Autodesk Inventor part; units mm, degrees
(part 2 of 2)
  spline S121 degree 2 poles (15.6602, 13.1424) (15.6885, 13.0846) (15.7439, 12.8774) (15.7439, 12.7846) knots 0 0 0 1 2 2 2
  spline S122 degree 2 poles (15.7439, 12.7846) (15.7439, 12.5888) (15.5368, 12.368) (15.3602, 12.368) knots 0 0 0 1 2 2 2
  spline S123 degree 2 poles (15.3602, 12.368) (15.2775, 12.368) (15.1394, 12.4065) (15.0805, 12.4405) knots 0 0 0 1 2 2 2
  spline S124 degree 2 poles (15.0805, 12.4405) (15.0194, 12.4744) (14.8994, 12.5729) (14.8417, 12.6273) knots 0 0 0 1 2 2 2
  spline S125 degree 2 poles (14.8417, 12.6273) (14.7454, 12.7156) (14.5394, 12.9318) (14.4794, 12.9963) knots 0 0 0 1 2 2 2
  line L109 (14.4794, 12.9963) -> (14.4794, 12.3103)
  line L110 (14.4794, 12.3103) -> (14.3175, 12.3103)
  line L111 (14.7975, 11.2246) -> (14.7975, 11.391)
  line L112 (14.7975, 11.391) -> (14.3175, 11.391)
  line L113 (14.3175, 11.391) -> (14.3175, 11.571)
  line L114 (14.3175, 11.571) -> (14.7975, 11.571)
  line L115 (14.7975, 11.571) -> (14.7975, 12.188)
  line L116 (14.7975, 12.188) -> (14.9945, 12.188)
  line L117 (14.9945, 12.188) -> (15.7145, 11.5631)
  line L118 (15.7145, 11.5631) -> (15.7145, 11.391)
  line L119 (15.7145, 11.391) -> (14.9481, 11.391)
  line L120 (14.9481, 11.391) -> (14.9481, 11.2246)
  line L121 (14.9481, 11.2246) -> (14.7975, 11.2246)
  line L122 (14.9481, 11.571) -> (15.4937, 11.571)
  line L123 (15.4937, 11.571) -> (14.9481, 12.0408)
  line L124 (14.9481, 12.0408) -> (14.9481, 11.571)
  spline S126 degree 2 poles (14.7613, 10.2284) (14.6605, 10.2284) (14.4884, 10.2929) (14.425, 10.3518) knots 0 0 0 1 2 2 2
  spline S127 degree 2 poles (14.425, 10.3518) (14.3616, 10.4106) (14.2881, 10.5861) (14.2881, 10.6948) knots 0 0 0 1 2 2 2
  spline S128 degree 2 poles (14.2881, 10.6948) (14.2881, 10.7944) (14.3322, 10.9891) (14.3673, 11.0604) knots 0 0 0 1 2 2 2
  line L125 (14.3673, 11.0604) -> (14.5654, 11.0604)
  line L126 (14.5654, 11.0604) -> (14.5654, 11.0469)
  spline S129 degree 2 poles (14.5654, 11.0469) (14.5496, 11.0253) (14.5088, 10.945) (14.4907, 10.8963) knots 0 0 0 1 2 2 2
  spline S130 degree 2 poles (14.4907, 10.8963) (14.4715, 10.8408) (14.4499, 10.7491) (14.4499, 10.6914) knots 0 0 0 1 2 2 2
  spline S131 degree 2 poles (14.4499, 10.6914) (14.4499, 10.6348) (14.4907, 10.5284) (14.5349, 10.4899) knots 0 0 0 1 2 2 2
  spline S132 degree 2 poles (14.5349, 10.4899) (14.5767, 10.4548) (14.6877, 10.4185) (14.7624, 10.4185) knots 0 0 0 1 2 2 2
  spline S133 degree 2 poles (14.7624, 10.4185) (14.8371, 10.4185) (14.9322, 10.4593) (14.9639, 10.4978) knots 0 0 0 1 2 2 2
  spline S134 degree 2 poles (14.9639, 10.4978) (14.999, 10.5374) (15.0284, 10.6552) (15.0284, 10.7265) knots 0 0 0 1 2 2 2
  spline S135 degree 2 poles (15.0284, 10.7265) (15.0284, 10.8035) (15.0047, 10.9563) (14.9945, 11.0027) knots 0 0 0 1 2 2 2
  line L127 (14.9945, 11.0027) -> (15.7145, 11.0027)
  line L128 (15.7145, 11.0027) -> (15.7145, 10.2363)
  line L129 (15.7145, 10.2363) -> (15.5503, 10.2363)
  line L130 (15.5503, 10.2363) -> (15.5503, 10.8227)
  line L131 (15.5503, 10.8227) -> (15.1779, 10.8227)
  spline S136 degree 2 poles (15.1779, 10.8227) (15.1824, 10.7887) (15.1858, 10.7231) (15.1858, 10.6959) knots 0 0 0 1 2 2 2
  spline S137 degree 2 poles (15.1858, 10.6959) (15.1858, 10.5884) (15.1507, 10.4401) (15.0986, 10.3721) knots 0 0 0 1 2 2 2
  spline S138 degree 2 poles (15.0986, 10.3721) (15.0466, 10.3031) (14.8881, 10.2284) (14.7613, 10.2284) knots 0 0 0 1 2 2 2
  spline S139 degree 2 poles (14.7703, 9.1438) (14.6628, 9.1438) (14.4805, 9.2151) (14.4194, 9.2751) knots 0 0 0 1 2 2 2
  spline S140 degree 2 poles (14.4194, 9.2751) (14.3549, 9.3374) (14.2881, 9.4936) (14.2881, 9.5876) knots 0 0 0 1 2 2 2
  spline S141 degree 2 poles (14.2881, 9.5876) (14.2881, 9.6816) (14.3515, 9.8367) (14.4149, 9.8955) knots 0 0 0 1 2 2 2
  spline S142 degree 2 poles (14.4149, 9.8955) (14.4907, 9.968) (14.7454, 10.0495) (14.9311, 10.0495) knots 0 0 0 1 2 2 2
  spline S143 degree 2 poles (14.9311, 10.0495) (15.1134, 10.0495) (15.4066, 9.9748) (15.5152, 9.8967) knots 0 0 0 1 2 2 2
  spline S144 degree 2 poles (15.5152, 9.8967) (15.6217, 9.8208) (15.7405, 9.5808) (15.7405, 9.4234) knots 0 0 0 1 2 2 2
  spline S145 degree 2 poles (15.7405, 9.4234) (15.7405, 9.377) (15.7315, 9.2955) (15.7213, 9.2649) knots 0 0 0 1 2 2 2
  line L132 (15.7213, 9.2649) -> (15.5413, 9.2649)
  line L133 (15.5413, 9.2649) -> (15.5413, 9.2729)
  spline S146 degree 2 poles (15.5413, 9.2729) (15.5549, 9.2989) (15.5786, 9.394) (15.5786, 9.4483) knots 0 0 0 1 2 2 2
  spline S147 degree 2 poles (15.5786, 9.4483) (15.5786, 9.6227) (15.3432, 9.8367) (15.1122, 9.857) knots 0 0 0 1 2 2 2
  spline S148 degree 2 poles (15.1122, 9.857) (15.1586, 9.7902) (15.2096, 9.6499) (15.2096, 9.5661) knots 0 0 0 1 2 2 2
  spline S149 degree 2 poles (15.2096, 9.5661) (15.2096, 9.4846) (15.1768, 9.3623) (15.1269, 9.2955) knots 0 0 0 1 2 2 2
  spline S150 degree 2 poles (15.1269, 9.2955) (15.0692, 9.2185) (14.8903, 9.1438) (14.7703, 9.1438) knots 0 0 0 1 2 2 2
  spline S151 degree 2 poles (14.7624, 9.334) (14.8484, 9.334) (14.9651, 9.3793) (15.0058, 9.4291) knots 0 0 0 1 2 2 2
  spline S152 degree 2 poles (15.0058, 9.4291) (15.0352, 9.4665) (15.0545, 9.5593) (15.0545, 9.608) knots 0 0 0 1 2 2 2
  spline S153 degree 2 poles (15.0545, 9.608) (15.0545, 9.6736) (15.0149, 9.797) (14.9775, 9.857) knots 0 0 0 1 2 2 2
  spline S154 degree 2 poles (14.9775, 9.857) (14.9571, 9.8582) (14.9186, 9.8604) (14.8892, 9.8604) knots 0 0 0 1 2 2 2
  spline S155 degree 2 poles (14.8892, 9.8604) (14.7443, 9.8604) (14.5666, 9.8038) (14.5201, 9.7608) knots 0 0 0 1 2 2 2
  spline S156 degree 2 poles (14.5201, 9.7608) (14.476, 9.7212) (14.4409, 9.6351) (14.4409, 9.5865) knots 0 0 0 1 2 2 2
  spline S157 degree 2 poles (14.4409, 9.5865) (14.4409, 9.4733) (14.6016, 9.334) (14.7624, 9.334) knots 0 0 0 1 2 2 2
  line L134 (15.5051, 8.1012) -> (14.3175, 8.7057)
  line L135 (14.3175, 8.7057) -> (14.3175, 8.9049)
  line L136 (14.3175, 8.9049) -> (15.5503, 8.2664)
  line L137 (15.5503, 8.2664) -> (15.5503, 8.9876)
  line L138 (15.5503, 8.9876) -> (15.7145, 8.9876)
  line L139 (15.7145, 8.9876) -> (15.7145, 8.1012)
  line L140 (15.7145, 8.1012) -> (15.5051, 8.1012)
  spline S158 degree 2 poles (15.016, 7.0608) (14.6401, 7.0608) (14.2881, 7.2793) (14.2881, 7.5068) knots 0 0 0 1 2 2 2
  spline S159 degree 2 poles (14.2881, 7.5068) (14.2881, 7.7378) (14.6469, 7.954) (15.0149, 7.954) knots 0 0 0 1 2 2 2
  spline S160 degree 2 poles (15.0149, 7.954) (15.393, 7.954) (15.7428, 7.7355) (15.7428, 7.5068) knots 0 0 0 1 2 2 2
  spline S161 degree 2 poles (15.7428, 7.5068) (15.7428, 7.277) (15.3805, 7.0608) (15.016, 7.0608) knots 0 0 0 1 2 2 2
  spline S162 degree 2 poles (14.5903, 7.3008) (14.6594, 7.2736) (14.8722, 7.251) (15.016, 7.251) knots 0 0 0 1 2 2 2
  spline S163 degree 2 poles (15.016, 7.251) (15.1598, 7.251) (15.3715, 7.2736) (15.4428, 7.3019) knots 0 0 0 1 2 2 2
  spline S164 degree 2 poles (15.4428, 7.3019) (15.5141, 7.3302) (15.5877, 7.4287) (15.5877, 7.5068) knots 0 0 0 1 2 2 2
  spline S165 degree 2 poles (15.5877, 7.5068) (15.5877, 7.5849) (15.5141, 7.6857) (15.4405, 7.7151) knots 0 0 0 1 2 2 2
  spline S166 degree 2 poles (15.4405, 7.7151) (15.3692, 7.7434) (15.1518, 7.7638) (15.0149, 7.7638) knots 0 0 0 1 2 2 2
  spline S167 degree 2 poles (15.0149, 7.7638) (14.8677, 7.7638) (14.6707, 7.7457) (14.5937, 7.7162) knots 0 0 0 1 2 2 2
  spline S168 degree 2 poles (14.5937, 7.7162) (14.5213, 7.6891) (14.4432, 7.5883) (14.4432, 7.5068) knots 0 0 0 1 2 2 2
  spline S169 degree 2 poles (14.4432, 7.5068) (14.4432, 7.4298) (14.5167, 7.3291) (14.5903, 7.3008) knots 0 0 0 1 2 2 2
  spline S170 degree 2 poles (15.582, 6.5049) (15.582, 6.5559) (15.5571, 6.6566) (15.5379, 6.7053) knots 0 0 0 1 2 2 2
  spline S171 degree 2 poles (15.5379, 6.7053) (15.5186, 6.7506) (15.4779, 6.8174) (15.4598, 6.8434) knots 0 0 0 1 2 2 2
  line L141 (15.4598, 6.8434) -> (15.4598, 6.8547)
  line L142 (15.4598, 6.8547) -> (15.6579, 6.8547)
  spline S172 degree 2 poles (15.6579, 6.8547) (15.6907, 6.7936) (15.7439, 6.5842) (15.7439, 6.4902) knots 0 0 0 1 2 2 2
  spline S173 degree 2 poles (15.7439, 6.4902) (15.7439, 6.3951) (15.7054, 6.2536) (15.6647, 6.1958) knots 0 0 0 1 2 2 2
  spline S174 degree 2 poles (15.6647, 6.1958) (15.6205, 6.1347) (15.4926, 6.0713) (15.4066, 6.0713) knots 0 0 0 1 2 2 2
  spline S175 degree 2 poles (15.4066, 6.0713) (15.2911, 6.0713) (15.1168, 6.223) (15.0941, 6.3294) knots 0 0 0 1 2 2 2
  line L143 (15.0941, 6.3294) -> (15.0805, 6.3294)
  spline S176 degree 2 poles (15.0805, 6.3294) (15.0715, 6.2853) (15.0307, 6.1845) (14.99, 6.1415) knots 0 0 0 1 2 2 2
  spline S177 degree 2 poles (14.99, 6.1415) (14.9503, 6.0985) (14.8235, 6.0441) (14.7318, 6.0441) knots 0 0 0 1 2 2 2
  spline S178 degree 2 poles (14.7318, 6.0441) (14.6379, 6.0441) (14.4783, 6.1087) (14.4171, 6.1675) knots 0 0 0 1 2 2 2
  spline S179 degree 2 poles (14.4171, 6.1675) (14.3537, 6.2287) (14.2881, 6.4019) (14.2881, 6.5117) knots 0 0 0 1 2 2 2
  spline S180 degree 2 poles (14.2881, 6.5117) (14.2881, 6.617) (14.339, 6.823) (14.3741, 6.8932) knots 0 0 0 1 2 2 2
  line L144 (14.3741, 6.8932) -> (14.5722, 6.8932)
  line L145 (14.5722, 6.8932) -> (14.5722, 6.8796)
  spline S181 degree 2 poles (14.5722, 6.8796) (14.5292, 6.8208) (14.4499, 6.6215) (14.4499, 6.523) knots 0 0 0 1 2 2 2
  spline S182 degree 2 poles (14.4499, 6.523) (14.4499, 6.4653) (14.4862, 6.3498) (14.5281, 6.3113) knots 0 0 0 1 2 2 2
  spline S183 degree 2 poles (14.5281, 6.3113) (14.57, 6.274) (14.6696, 6.2343) (14.7454, 6.2343) knots 0 0 0 1 2 2 2
  spline S184 degree 2 poles (14.7454, 6.2343) (14.8213, 6.2343) (14.9198, 6.2785) (14.9481, 6.3181) knots 0 0 0 1 2 2 2
  spline S185 degree 2 poles (14.9481, 6.3181) (14.9764, 6.3577) (14.9979, 6.4653) (14.9979, 6.5287) knots 0 0 0 1 2 2 2
  line L146 (14.9979, 6.5287) -> (14.9979, 6.6079)
  line L147 (14.9979, 6.6079) -> (15.153, 6.6079)
  line L148 (15.153, 6.6079) -> (15.153, 6.5457)
  spline S186 degree 2 poles (15.153, 6.5457) (15.153, 6.42) (15.273, 6.2615) (15.3873, 6.2615) knots 0 0 0 1 2 2 2
  spline S187 degree 2 poles (15.3873, 6.2615) (15.4405, 6.2615) (15.5164, 6.3023) (15.539, 6.3351) knots 0 0 0 1 2 2 2
  spline S188 degree 2 poles (15.539, 6.3351) (15.5628, 6.3702) (15.582, 6.4562) (15.582, 6.5049) knots 0 0 0 1 2 2 2
  line L149 (12.0174, 19.3553) -> (12.0174, 19.5319)
  line L150 (12.0174, 19.5319) -> (12.1238, 19.5319)
  spline S189 degree 2 poles (12.1238, 19.5319) (12.0898, 19.5726) (12.0445, 19.6326) (12.0253, 19.6734) knots 0 0 0 1 2 2 2
  spline S190 degree 2 poles (12.0253, 19.6734) (12.0072, 19.7107) (11.9879, 19.7911) (11.9879, 19.8443) knots 0 0 0 1 2 2 2
  spline S191 degree 2 poles (11.9879, 19.8443) (11.9879, 19.9304) (12.0593, 20.0753) (12.1283, 20.1262) knots 0 0 0 1 2 2 2
  spline S192 degree 2 poles (12.1283, 20.1262) (12.1974, 20.1772) (12.4011, 20.2338) (12.5336, 20.2338) knots 0 0 0 1 2 2 2
  spline S193 degree 2 poles (12.5336, 20.2338) (12.6717, 20.2338) (12.8732, 20.1625) (12.9491, 20.1002) knots 0 0 0 1 2 2 2
  spline S194 degree 2 poles (12.9491, 20.1002) (13.017, 20.0425) (13.0951, 19.8806) (13.0951, 19.7911) knots 0 0 0 1 2 2 2
  spline S195 degree 2 poles (13.0951, 19.7911) (13.0951, 19.713) (13.06, 19.5964) (13.0238, 19.5319) knots 0 0 0 1 2 2 2
  line L151 (13.0238, 19.5319) -> (13.4766, 19.5319)
  line L152 (13.4766, 19.5319) -> (13.4766, 19.3553)
  line L153 (13.4766, 19.3553) -> (12.0174, 19.3553)
  line L154 (12.2721, 19.5319) -> (12.8778, 19.5319)
  spline S196 degree 2 poles (12.8778, 19.5319) (12.9095, 19.5975) (12.9332, 19.7017) (12.9332, 19.7617) knots 0 0 0 1 2 2 2
  spline S197 degree 2 poles (12.9332, 19.7617) (12.9332, 19.8975) (12.7295, 20.0515) (12.537, 20.0515) knots 0 0 0 1 2 2 2
  spline S198 degree 2 poles (12.537, 20.0515) (12.3513, 20.0515) (12.1555, 19.9338) (12.1555, 19.8036) knots 0 0 0 1 2 2 2
  spline S199 degree 2 poles (12.1555, 19.8036) (12.1555, 19.7345) (12.2189, 19.5941) (12.2721, 19.5319) knots 0 0 0 1 2 2 2
  spline S200 degree 2 poles (12.1283, 18.5153) (12.1125, 18.5368) (12.0559, 18.6092) (12.0389, 18.6432) knots 0 0 0 1 2 2 2
  spline S201 degree 2 poles (12.0389, 18.6432) (12.014, 18.6896) (11.9879, 18.7768) (11.9879, 18.856) knots 0 0 0 1 2 2 2
  spline S202 degree 2 poles (11.9879, 18.856) (11.9879, 18.9205) (12.0366, 19.0372) (12.0808, 19.0813) knots 0 0 0 1 2 2 2
  spline S203 degree 2 poles (12.0808, 19.0813) (12.1238, 19.1232) (12.2506, 19.1741) (12.3208, 19.1741) knots 0 0 0 1 2 2 2
  spline S204 degree 2 poles (12.3208, 19.1741) (12.4295, 19.1741) (12.5834, 19.0824) (12.6276, 18.9828) knots 0 0 0 1 2 2 2
  spline S205 degree 2 poles (12.6276, 18.9828) (12.6683, 18.8945) (12.6989, 18.6545) (12.7068, 18.5153) knots 0 0 0 1 2 2 2
  line L155 (12.7068, 18.5153) -> (12.7408, 18.5153)
  spline S206 degree 2 poles (12.7408, 18.5153) (12.8019, 18.5153) (12.8778, 18.5526) (12.8993, 18.5866) knots 0 0 0 1 2 2 2
  spline S207 degree 2 poles (12.8993, 18.5866) (12.9208, 18.6205) (12.9344, 18.7179) (12.9344, 18.77) knots 0 0 0 1 2 2 2
  spline S208 degree 2 poles (12.9344, 18.77) (12.9344, 18.8311) (12.8981, 18.9964) (12.863, 19.079) knots 0 0 0 1 2 2 2
  line L156 (12.863, 19.079) -> (12.863, 19.0892)
  line L157 (12.863, 19.0892) -> (13.043, 19.0892)
  spline S209 degree 2 poles (13.043, 19.0892) (13.0566, 19.0406) (13.0906, 18.8583) (13.0906, 18.7688) knots 0 0 0 1 2 2 2
  spline S210 degree 2 poles (13.0906, 18.7688) (13.0906, 18.6602) (13.0566, 18.5119) (13.0125, 18.453) knots 0 0 0 1 2 2 2
  spline S211 degree 2 poles (13.0125, 18.453) (12.9695, 18.3953) (12.8325, 18.3387) (12.734, 18.3387) knots 0 0 0 1 2 2 2
  line L158 (12.734, 18.3387) -> (12.0174, 18.3387)
  line L159 (12.0174, 18.3387) -> (12.0174, 18.5153)
  line L160 (12.0174, 18.5153) -> (12.1283, 18.5153)
  line L161 (12.2755, 18.5153) -> (12.5664, 18.5153)
  spline S212 degree 2 poles (12.5664, 18.5153) (12.5608, 18.5787) (12.5415, 18.77) (12.5234, 18.83) knots 0 0 0 1 2 2 2
  spline S213 degree 2 poles (12.5234, 18.83) (12.5019, 18.9002) (12.4125, 18.9919) (12.3332, 18.9919) knots 0 0 0 1 2 2 2
  spline S214 degree 2 poles (12.3332, 18.9919) (12.2427, 18.9919) (12.151, 18.89) (12.151, 18.7926) knots 0 0 0 1 2 2 2
  spline S215 degree 2 poles (12.151, 18.7926) (12.151, 18.71) (12.2223, 18.5741) (12.2755, 18.5153) knots 0 0 0 1 2 2 2
  line L162 (12.8766, 17.5349) -> (12.8766, 17.5439)
  spline S216 degree 2 poles (12.8766, 17.5439) (12.8823, 17.5643) (12.8846, 17.6085) (12.8846, 17.639) knots 0 0 0 1 2 2 2
  spline S217 degree 2 poles (12.8846, 17.639) (12.8846, 17.7103) (12.8223, 17.8507) (12.7612, 17.9141) knots 0 0 0 1 2 2 2
  line L163 (12.7612, 17.9141) -> (12.0174, 17.9141)
  line L164 (12.0174, 17.9141) -> (12.0174, 18.0907)
  line L165 (12.0174, 18.0907) -> (13.0657, 18.0907)
  line L166 (13.0657, 18.0907) -> (13.0657, 17.9141)
  line L167 (13.0657, 17.9141) -> (12.9095, 17.9141)
  spline S218 degree 2 poles (12.9095, 17.9141) (12.9955, 17.8179) (13.0657, 17.6741) (13.0657, 17.6062) knots 0 0 0 1 2 2 2
  spline S219 degree 2 poles (13.0657, 17.6062) (13.0657, 17.579) (13.0634, 17.5519) (13.06, 17.5349) knots 0 0 0 1 2 2 2
  line L168 (13.06, 17.5349) -> (12.8766, 17.5349)
  spline S220 degree 2 poles (11.9925, 17.1149) (11.9925, 17.2201) (12.0491, 17.4024) (12.0808, 17.4624) knots 0 0 0 1 2 2 2
  line L169 (12.0808, 17.4624) -> (12.2789, 17.4624)
  line L170 (12.2789, 17.4624) -> (12.2789, 17.4534)
  spline S221 degree 2 poles (12.2789, 17.4534) (12.2608, 17.4307) (12.2178, 17.3696) (12.194, 17.3186) knots 0 0 0 1 2 2 2
  spline S222 degree 2 poles (12.194, 17.3186) (12.1725, 17.2745) (12.1408, 17.1658) (12.1408, 17.1081) knots 0 0 0 1 2 2 2
  spline S223 degree 2 poles (12.1408, 17.1081) (12.1408, 17.0662) (12.16, 16.97) (12.1759, 16.9473) knots 0 0 0 1 2 2 2
  spline S224 degree 2 poles (12.1759, 16.9473) (12.1974, 16.9145) (12.2461, 16.8851) (12.2959, 16.8851) knots 0 0 0 1 2 2 2
  spline S225 degree 2 poles (12.2959, 16.8851) (12.3581, 16.8851) (12.4227, 16.953) (12.4442, 17.0401) knots 0 0 0 1 2 2 2
  spline S226 degree 2 poles (12.4442, 17.0401) (12.4521, 17.0741) (12.4747, 17.1828) (12.4872, 17.2292) knots 0 0 0 1 2 2 2
  spline S227 degree 2 poles (12.4872, 17.2292) (12.5223, 17.3492) (12.6672, 17.4579) (12.7702, 17.4579) knots 0 0 0 1 2 2 2
  spline S228 degree 2 poles (12.7702, 17.4579) (12.9129, 17.4579) (13.0906, 17.2439) (13.0906, 17.0673) knots 0 0 0 1 2 2 2
  spline S229 degree 2 poles (13.0906, 17.0673) (13.0906, 16.9801) (13.0476, 16.8035) (13.0147, 16.7435) knots 0 0 0 1 2 2 2
  line L171 (13.0147, 16.7435) -> (12.8257, 16.7435)
  line L172 (12.8257, 16.7435) -> (12.8257, 16.7526)
  spline S230 degree 2 poles (12.8257, 16.7526) (12.88, 16.8205) (12.9423, 16.9858) (12.9423, 17.0707) knots 0 0 0 1 2 2 2
  spline S231 degree 2 poles (12.9423, 17.0707) (12.9423, 17.1579) (12.8687, 17.2779) (12.7951, 17.2779) knots 0 0 0 1 2 2 2
  spline S232 degree 2 poles (12.7951, 17.2779) (12.7283, 17.2779) (12.6638, 17.2066) (12.6434, 17.1273) knots 0 0 0 1 2 2 2
  spline S233 degree 2 poles (12.6434, 17.1273) (12.6332, 17.0888) (12.6129, 16.9915) (12.6004, 16.9383) knots 0 0 0 1 2 2 2
  spline S234 degree 2 poles (12.6004, 16.9383) (12.571, 16.8228) (12.4362, 16.705) (12.3196, 16.705) knots 0 0 0 1 2 2 2
  spline S235 degree 2 poles (12.3196, 16.705) (12.2517, 16.705) (12.1317, 16.7583) (12.0876, 16.8103) knots 0 0 0 1 2 2 2
  spline S236 degree 2 poles (12.0876, 16.8103) (12.0411, 16.8658) (11.9925, 17.0073) (11.9925, 17.1149) knots 0 0 0 1 2 2 2
  line L173 (12.0174, 15.7179) -> (12.0174, 15.8945)
  line L174 (12.0174, 15.8945) -> (12.6151, 15.8945)
  spline S237 degree 2 poles (12.6151, 15.8945) (12.6876, 15.8945) (12.8121, 15.9081) (12.8495, 15.9284) knots 0 0 0 1 2 2 2
  spline S238 degree 2 poles (12.8495, 15.9284) (12.8891, 15.9499) (12.9276, 16.0269) (12.9276, 16.0926) knots 0 0 0 1 2 2 2
  spline S239 degree 2 poles (12.9276, 16.0926) (12.9276, 16.1582) (12.8574, 16.2975) (12.8008, 16.3643) knots 0 0 0 1 2 2 2
  line L175 (12.8008, 16.3643) -> (12.0174, 16.3643)
  line L176 (12.0174, 16.3643) -> (12.0174, 16.5409)
  line L177 (12.0174, 16.5409) -> (13.4766, 16.5409)
  line L178 (13.4766, 16.5409) -> (13.4766, 16.3643)
  line L179 (13.4766, 16.3643) -> (12.9491, 16.3643)
  spline S240 degree 2 poles (12.9491, 16.3643) (13.0204, 16.285) (13.0951, 16.1322) (13.0951, 16.0462) knots 0 0 0 1 2 2 2
  spline S241 degree 2 poles (13.0951, 16.0462) (13.0951, 15.8922) (12.8913, 15.7179) (12.6978, 15.7179) knots 0 0 0 1 2 2 2
  line L180 (12.6978, 15.7179) -> (12.0174, 15.7179)
  line L181 (12.0174, 15.2899) -> (12.0174, 15.4665)
  line L182 (12.0174, 15.4665) -> (13.0657, 15.4665)
  line L183 (13.0657, 15.4665) -> (13.0657, 15.2899)
  line L184 (13.0657, 15.2899) -> (12.0174, 15.2899)
  line L185 (13.24, 15.2775) -> (13.24, 15.4779)
  line L186 (13.24, 15.4779) -> (13.4234, 15.4779)
  line L187 (13.4234, 15.4779) -> (13.4234, 15.2775)
  line L188 (13.4234, 15.2775) -> (13.24, 15.2775)
  line L189 (12.0174, 14.8507) -> (12.0174, 15.0273)
  line L190 (12.0174, 15.0273) -> (13.4766, 15.0273)
  line L191 (13.4766, 15.0273) -> (13.4766, 14.8507)
  line L192 (13.4766, 14.8507) -> (12.0174, 14.8507)
  spline S242 degree 2 poles (12.5698, 13.7129) (12.3072, 13.7129) (11.997, 13.9631) (11.997, 14.1544) knots 0 0 0 1 2 2 2
  spline S243 degree 2 poles (11.997, 14.1544) (11.997, 14.2326) (12.0332, 14.3526) (12.0706, 14.4148) knots 0 0 0 1 2 2 2
  line L193 (12.0706, 14.4148) -> (11.6313, 14.4148)
  line L194 (11.6313, 14.4148) -> (11.6313, 14.5914)
  line L195 (11.6313, 14.5914) -> (13.0657, 14.5914)
  line L196 (13.0657, 14.5914) -> (13.0657, 14.4148)
  line L197 (13.0657, 14.4148) -> (12.9559, 14.4148)
  spline S244 degree 2 poles (12.9559, 14.4148) (13.0159, 14.3492) (13.0951, 14.1884) (13.0951, 14.0944) knots 0 0 0 1 2 2 2
  spline S245 degree 2 poles (13.0951, 14.0944) (13.0951, 13.9144) (12.8098, 13.7129) (12.5698, 13.7129) knots 0 0 0 1 2 2 2
  spline S246 degree 2 poles (12.5495, 13.8952) (12.7295, 13.8952) (12.9276, 14.0095) (12.9276, 14.1375) knots 0 0 0 1 2 2 2
  spline S247 degree 2 poles (12.9276, 14.1375) (12.9276, 14.2122) (12.8608, 14.3526) (12.8087, 14.4148) knots 0 0 0 1 2 2 2
  line L198 (12.8087, 14.4148) -> (12.2132, 14.4148)
  spline S248 degree 2 poles (12.2132, 14.4148) (12.1804, 14.3458) (12.1555, 14.2473) (12.1555, 14.1839) knots 0 0 0 1 2 2 2
  spline S249 degree 2 poles (12.1555, 14.1839) (12.1555, 14.0469) (12.357, 13.8952) (12.5495, 13.8952) knots 0 0 0 1 2 2 2
  spline S250 degree 2 poles (12.1283, 12.9454) (12.1125, 12.9669) (12.0559, 13.0393) (12.0389, 13.0733) knots 0 0 0 1 2 2 2
  spline S251 degree 2 poles (12.0389, 13.0733) (12.014, 13.1197) (11.9879, 13.2069) (11.9879, 13.2861) knots 0 0 0 1 2 2 2
  spline S252 degree 2 poles (11.9879, 13.2861) (11.9879, 13.3507) (12.0366, 13.4673) (12.0808, 13.5114) knots 0 0 0 1 2 2 2
  spline S253 degree 2 poles (12.0808, 13.5114) (12.1238, 13.5533) (12.2506, 13.6043) (12.3208, 13.6043) knots 0 0 0 1 2 2 2
  spline S254 degree 2 poles (12.3208, 13.6043) (12.4295, 13.6043) (12.5834, 13.5126) (12.6276, 13.4129) knots 0 0 0 1 2 2 2
  spline S255 degree 2 poles (12.6276, 13.4129) (12.6683, 13.3246) (12.6989, 13.0846) (12.7068, 12.9454) knots 0 0 0 1 2 2 2
  line L199 (12.7068, 12.9454) -> (12.7408, 12.9454)
  spline S256 degree 2 poles (12.7408, 12.9454) (12.8019, 12.9454) (12.8778, 12.9827) (12.8993, 13.0167) knots 0 0 0 1 2 2 2
  spline S257 degree 2 poles (12.8993, 13.0167) (12.9208, 13.0507) (12.9344, 13.148) (12.9344, 13.2001) knots 0 0 0 1 2 2 2
  spline S258 degree 2 poles (12.9344, 13.2001) (12.9344, 13.2612) (12.8981, 13.4265) (12.863, 13.5092) knots 0 0 0 1 2 2 2
  line L200 (12.863, 13.5092) -> (12.863, 13.5193)
  line L201 (12.863, 13.5193) -> (13.043, 13.5193)
  spline S259 degree 2 poles (13.043, 13.5193) (13.0566, 13.4707) (13.0906, 13.2884) (13.0906, 13.199) knots 0 0 0 1 2 2 2
  spline S260 degree 2 poles (13.0906, 13.199) (13.0906, 13.0903) (13.0566, 12.942) (13.0125, 12.8831) knots 0 0 0 1 2 2 2
  spline S261 degree 2 poles (13.0125, 12.8831) (12.9695, 12.8254) (12.8325, 12.7688) (12.734, 12.7688) knots 0 0 0 1 2 2 2
  line L202 (12.734, 12.7688) -> (12.0174, 12.7688)
  line L203 (12.0174, 12.7688) -> (12.0174, 12.9454)
  line L204 (12.0174, 12.9454) -> (12.1283, 12.9454)
  line L205 (12.2755, 12.9454) -> (12.5664, 12.9454)
  spline S262 degree 2 poles (12.5664, 12.9454) (12.5608, 13.0088) (12.5415, 13.2001) (12.5234, 13.2601) knots 0 0 0 1 2 2 2
  spline S263 degree 2 poles (12.5234, 13.2601) (12.5019, 13.3303) (12.4125, 13.422) (12.3332, 13.422) knots 0 0 0 1 2 2 2
  spline S264 degree 2 poles (12.3332, 13.422) (12.2427, 13.422) (12.151, 13.3201) (12.151, 13.2227) knots 0 0 0 1 2 2 2
  spline S265 degree 2 poles (12.151, 13.2227) (12.151, 13.1401) (12.2223, 13.0042) (12.2755, 12.9454) knots 0 0 0 1 2 2 2
  spline S266 degree 2 poles (11.997, 12.2039) (11.997, 12.3476) (12.1611, 12.5095) (12.3389, 12.5095) knots 0 0 0 1 2 2 2
  line L206 (12.3389, 12.5095) -> (12.9196, 12.5095)
  line L207 (12.9196, 12.5095) -> (12.9196, 12.6284)
  line L208 (12.9196, 12.6284) -> (13.0657, 12.6284)
  line L209 (13.0657, 12.6284) -> (13.0657, 12.5095)
  line L210 (13.0657, 12.5095) -> (13.3668, 12.5095)
  line L211 (13.3668, 12.5095) -> (13.3668, 12.3329)
  line L212 (13.3668, 12.3329) -> (13.0657, 12.3329)
  line L213 (13.0657, 12.3329) -> (13.0657, 12.008)
  line L214 (13.0657, 12.008) -> (12.9196, 12.008)
  line L215 (12.9196, 12.008) -> (12.9196, 12.3329)
  line L216 (12.9196, 12.3329) -> (12.4204, 12.3329)
  spline S267 degree 2 poles (12.4204, 12.3329) (12.3411, 12.3329) (12.254, 12.3273) (12.2166, 12.308) knots 0 0 0 1 2 2 2
  spline S268 degree 2 poles (12.2166, 12.308) (12.1838, 12.2922) (12.151, 12.2208) (12.151, 12.1597) knots 0 0 0 1 2 2 2
  spline S269 degree 2 poles (12.151, 12.1597) (12.151, 12.1167) (12.177, 12.0363) (12.1849, 12.0182) knots 0 0 0 1 2 2 2
  line L217 (12.1849, 12.0182) -> (12.1849, 12.008)
  line L218 (12.1849, 12.008) -> (12.0264, 12.008)
  spline S270 degree 2 poles (12.0264, 12.008) (12.0128, 12.0578) (11.997, 12.1597) (11.997, 12.2039) knots 0 0 0 1 2 2 2
  spline S271 degree 2 poles (11.9936, 11.4227) (11.9936, 11.674) (12.2755, 11.9503) (12.5359, 11.9503) knots 0 0 0 1 2 2 2
  spline S272 degree 2 poles (12.5359, 11.9503) (12.7917, 11.9503) (13.0951, 11.682) (13.0951, 11.4657) knots 0 0 0 1 2 2 2
  spline S273 degree 2 poles (13.0951, 11.4657) (13.0951, 11.3684) (13.0385, 11.2178) (12.9785, 11.1623) knots 0 0 0 1 2 2 2
  spline S274 degree 2 poles (12.9785, 11.1623) (12.9185, 11.1057) (12.7453, 11.0457) (12.6196, 11.0457) knots 0 0 0 1 2 2 2
  line L219 (12.6196, 11.0457) -> (12.5234, 11.0457)
  line L220 (12.5234, 11.0457) -> (12.5234, 11.7714)
  spline S275 degree 2 poles (12.5234, 11.7714) (12.3411, 11.7714) (12.1476, 11.588) (12.1476, 11.425) knots 0 0 0 1 2 2 2
  spline S276 degree 2 poles (12.1476, 11.425) (12.1476, 11.3672) (12.1736, 11.2552) (12.194, 11.2099) knots 0 0 0 1 2 2 2
  spline S277 degree 2 poles (12.194, 11.2099) (12.2166, 11.1623) (12.2562, 11.0967) (12.2744, 11.0752) knots 0 0 0 1 2 2 2
  line L221 (12.2744, 11.0752) -> (12.2744, 11.065)
  line L222 (12.2744, 11.065) -> (12.0819, 11.065)
  spline S278 degree 2 poles (12.0819, 11.065) (12.0694, 11.0955) (12.0332, 11.1884) (12.023, 11.2246) knots 0 0 0 1 2 2 2
  spline S279 degree 2 poles (12.023, 11.2246) (12.0083, 11.2755) (11.9936, 11.3593) (11.9936, 11.4227) knots 0 0 0 1 2 2 2
  spline S280 degree 2 poles (12.6581, 11.2178) (12.7295, 11.2201) (12.8336, 11.2495) (12.8687, 11.2778) knots 0 0 0 1 2 2 2
  spline S281 degree 2 poles (12.8687, 11.2778) (12.9083, 11.3084) (12.9502, 11.4046) (12.9502, 11.4759) knots 0 0 0 1 2 2 2
  spline S282 degree 2 poles (12.9502, 11.4759) (12.9502, 11.5461) (12.9083, 11.6446) (12.8676, 11.6854) knots 0 0 0 1 2 2 2
  spline S283 degree 2 poles (12.8676, 11.6854) (12.8257, 11.725) (12.7249, 11.7657) (12.6581, 11.7714) knots 0 0 0 1 2 2 2
  line L223 (12.6581, 11.7714) -> (12.6581, 11.2178)
  line L224 (12.0174, 10.6869) -> (12.0174, 10.8635)
  line L225 (12.0174, 10.8635) -> (13.4766, 10.8635)
  line L226 (13.4766, 10.8635) -> (13.4766, 10.6869)
  line L227 (13.4766, 10.6869) -> (12.0174, 10.6869)
  line L228 (12.0174, 10.1536) -> (12.0174, 10.3778)
  line L229 (12.0174, 10.3778) -> (12.2845, 10.3778)
  line L230 (12.2845, 10.3778) -> (12.2845, 10.1536)
  line L231 (12.2845, 10.1536) -> (12.0174, 10.1536)
  spline S284 degree 2 poles (11.9936, 9.4291) (11.9936, 9.5378) (12.0604, 9.7178) (12.1283, 9.7823) knots 0 0 0 1 2 2 2
  spline S285 degree 2 poles (12.1283, 9.7823) (12.1951, 9.8468) (12.4011, 9.9182) (12.5393, 9.9182) knots 0 0 0 1 2 2 2
  spline S286 degree 2 poles (12.5393, 9.9182) (12.6774, 9.9182) (12.8789, 9.8446) (12.9468, 9.7823) knots 0 0 0 1 2 2 2
  spline S287 degree 2 poles (12.9468, 9.7823) (13.0159, 9.72) (13.0895, 9.5355) (13.0895, 9.4291) knots 0 0 0 1 2 2 2
  spline S288 degree 2 poles (13.0895, 9.4291) (13.0895, 9.3431) (13.0408, 9.1823) (13.0091, 9.12) knots 0 0 0 1 2 2 2
  line L232 (13.0091, 9.12) -> (12.811, 9.12)
  line L233 (12.811, 9.12) -> (12.811, 9.1302)
  spline S289 degree 2 poles (12.811, 9.1302) (12.8268, 9.1495) (12.8676, 9.2083) (12.8891, 9.2502) knots 0 0 0 1 2 2 2
  spline S290 degree 2 poles (12.8891, 9.2502) (12.9072, 9.2876) (12.9355, 9.3872) (12.9355, 9.4325) knots 0 0 0 1 2 2 2
  spline S291 degree 2 poles (12.9355, 9.4325) (12.9355, 9.5695) (12.7283, 9.7359) (12.5393, 9.7359) knots 0 0 0 1 2 2 2
  spline S292 degree 2 poles (12.5393, 9.7359) (12.3547, 9.7359) (12.1476, 9.5751) (12.1476, 9.4325) knots 0 0 0 1 2 2 2
  spline S293 degree 2 poles (12.1476, 9.4325) (12.1476, 9.3465) (12.2189, 9.1902) (12.2744, 9.1302) knots 0 0 0 1 2 2 2
  line L234 (12.2744, 9.1302) -> (12.2744, 9.12)
  line L235 (12.2744, 9.12) -> (12.0762, 9.12)
  spline S294 degree 2 poles (12.0762, 9.12) (12.0638, 9.1461) (12.0287, 9.2253) (12.0208, 9.257) knots 0 0 0 1 2 2 2
  spline S295 degree 2 poles (12.0208, 9.257) (12.0072, 9.3023) (11.9936, 9.3736) (11.9936, 9.4291) knots 0 0 0 1 2 2 2
  spline S296 degree 2 poles (12.5415, 8.0978) (12.2766, 8.0978) (11.9879, 8.3525) (11.9879, 8.5653) knots 0 0 0 1 2 2 2
  spline S297 degree 2 poles (11.9879, 8.5653) (11.9879, 8.7838) (12.2857, 9.034) (12.5415, 9.034) knots 0 0 0 1 2 2 2
  spline S298 degree 2 poles (12.5415, 9.034) (12.8042, 9.034) (13.0951, 8.7759) (13.0951, 8.5653) knots 0 0 0 1 2 2 2
  spline S299 degree 2 poles (13.0951, 8.5653) (13.0951, 8.3525) (12.8053, 8.0978) (12.5415, 8.0978) knots 0 0 0 1 2 2 2
  spline S300 degree 2 poles (12.5415, 8.28) (12.7453, 8.28) (12.9434, 8.4283) (12.9434, 8.5653) knots 0 0 0 1 2 2 2
  spline S301 degree 2 poles (12.9434, 8.5653) (12.9434, 8.7023) (12.7453, 8.8517) (12.5415, 8.8517) knots 0 0 0 1 2 2 2
  spline S302 degree 2 poles (12.5415, 8.8517) (12.3434, 8.8517) (12.1396, 8.7023) (12.1396, 8.5653) knots 0 0 0 1 2 2 2
  spline S303 degree 2 poles (12.1396, 8.5653) (12.1396, 8.4295) (12.34, 8.28) (12.5415, 8.28) knots 0 0 0 1 2 2 2
  line L236 (12.0174, 6.7279) -> (12.6242, 6.7279)
  spline S304 degree 2 poles (12.6242, 6.7279) (12.6966, 6.7279) (12.82, 6.7393) (12.854, 6.7574) knots 0 0 0 1 2 2 2
  spline S305 degree 2 poles (12.854, 6.7574) (12.8913, 6.7755) (12.9276, 6.8445) (12.9276, 6.9045) knots 0 0 0 1 2 2 2
  spline S306 degree 2 poles (12.9276, 6.9045) (12.9276, 6.9589) (12.8608, 7.0834) (12.7974, 7.1491) knots 0 0 0 1 2 2 2
  spline S307 degree 2 poles (12.7974, 7.1491) (12.7815, 7.1479) (12.7374, 7.1457) (12.7079, 7.1457) knots 0 0 0 1 2 2 2
  line L237 (12.7079, 7.1457) -> (12.0174, 7.1457)
  line L238 (12.0174, 7.1457) -> (12.0174, 7.3223)
  line L239 (12.0174, 7.3223) -> (12.6242, 7.3223)
  spline S308 degree 2 poles (12.6242, 7.3223) (12.6966, 7.3223) (12.82, 7.3336) (12.854, 7.3517) knots 0 0 0 1 2 2 2
  spline S309 degree 2 poles (12.854, 7.3517) (12.8913, 7.3698) (12.9276, 7.4389) (12.9276, 7.4989) knots 0 0 0 1 2 2 2
  spline S310 degree 2 poles (12.9276, 7.4989) (12.9276, 7.5555) (12.8563, 7.6812) (12.8008, 7.74) knots 0 0 0 1 2 2 2
  line L240 (12.8008, 7.74) -> (12.0174, 7.74)
  line L241 (12.0174, 7.74) -> (12.0174, 7.9166)
  line L242 (12.0174, 7.9166) -> (13.0657, 7.9166)
  line L243 (13.0657, 7.9166) -> (13.0657, 7.74)
  line L244 (13.0657, 7.74) -> (12.9502, 7.74)
  spline S311 degree 2 poles (12.9502, 7.74) (13.0193, 7.671) (13.0951, 7.5351) (13.0951, 7.4536) knots 0 0 0 1 2 2 2
  spline S312 degree 2 poles (13.0951, 7.4536) (13.0951, 7.3608) (13.0102, 7.217) (12.914, 7.1796) knots 0 0 0 1 2 2 2
  spline S313 degree 2 poles (12.914, 7.1796) (13.0034, 7.0993) (13.0951, 6.9476) (13.0951, 6.8593) knots 0 0 0 1 2 2 2
  spline S314 degree 2 poles (13.0951, 6.8593) (13.0951, 6.7913) (13.0532, 6.6804) (13.0057, 6.6396) knots 0 0 0 1 2 2 2
  spline S315 degree 2 poles (13.0057, 6.6396) (12.9581, 6.5977) (12.8155, 6.5513) (12.7079, 6.5513) knots 0 0 0 1 2 2 2
  line L245 (12.7079, 6.5513) -> (12.0174, 6.5513)
  line L246 (12.0174, 6.5513) -> (12.0174, 6.7279)
  point P0 (0, 0)
  constraints: 2 other
emboss "Emboss2" sketch "Sketch46" operation cut depth 1.27 direction (1, 0, 0)
body "Solid1"
body "Srf1"
